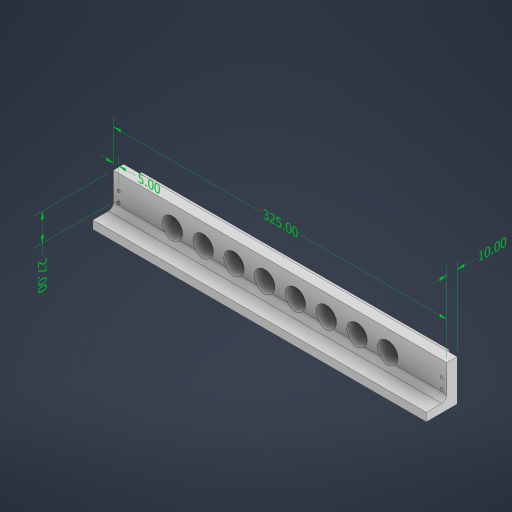
# Autodesk Inventor part: chessboard-base-1
Saved by Autodesk Inventor 2023 (Build 270158000, 158)
## iProperties
Created: 2023-12-20
Part Number: chessboard-base-1
Material: Generic
Document SubType Name: Modeling
Designer: hrush
Density: 1 g/cm^3
Appearance: Default
Author: hrush
Autodesk Inventor part; units mm, degrees
ref_plane "YZ Plane" through (0, 0, 0) normal (1, 0, 0) x (0, 1, 0)
ref_plane "XZ Plane" through (0, 0, 0) normal (0, 1, 0) x (-1, 0, 0)
ref_plane "XY Plane" through (0, 0, 0) normal (0, 0, 1) x (1, 0, 0)
sketch "Sketch1" plane through (0, 0, 0) normal (0, 1, 0) x (-1, 0, 0)
  line L0 (0, 0) -> (325, 0)
  line L1 (325, 0) -> (325, -10)
  line L2 (325, -10) -> (0, -10)
  line L3 (0, -10) -> (0, 0)
  dimension "d0" = 325
  dimension "d1" = 10
  constraints: 8 end point, 2 parallel, 1 horizontal, 1 perpendicular
  measures "d0" distance of L1.end L2.end
  measures "d1" distance of L0.end L1.end
extrude "Extrusion1" add sketch "Sketch1" along normal blind 40
sketch "Sketch4" plane through (-325, 0, 0) normal (0, 0, 1) x (1, 0, 0)
  line L0 (325, 0) -> (0, 0) projected
  line L1 (325, 0) -> (325, 40) projected
  line L2 (0, 0) -> (325, 0)
  line L3 (325, 0) -> (325, 8)
  line L4 (325, 8) -> (0, 8)
  line L5 (0, 8) -> (0, 0)
  dimension "d34" = 8
  constraints: 8 end point, 2 parallel, 1 horizontal, 1 perpendicular, 1 point on line
  measures "d34" distance of L3.end L2.end
extrude "Extrusion3" add sketch "Sketch4" along normal blind 20
sketch "Sketch5" plane through (-325, 40, 0) normal (0, 0, 1) x (1, 0, 0)
  circle A0 centre (320, -25) radius 1.5
  circle A1 centre (320, -15) radius 1.5
  line L0 (325, -32) -> (325, 0) projected
  line L1 (0, 0) -> (325, 0) projected
  circle A2 centre (5, -15) radius 1.5
  circle A3 centre (5, -25) radius 1.5
  line L2 (0, -32) -> (0, 0) projected
  point P0 (325, -40)
  point P1 (325, -27)
  point P2 (0, -27)
  dimension "d39" = 3
  dimension "d40" = 3
  dimension "d41" = 5
  dimension "d42" = 5
  dimension "d43" = 10
  dimension "d44" = 15
  dimension "d45" = 3
  dimension "d46" = 3
  dimension "d47" = 10
  dimension "d48" = 15
  dimension "d49" = 5
  dimension "d50" = 5
  constraints: 4 centre point
  measures "d39" diameter of A0
  measures "d40" diameter of A1
  measures "d41" distance from line of L0 A0.centre
  measures "d42" distance from line of L0 A1.centre
  measures "d43" distance of A0.centre A1.centre
  measures "d44" distance from line of L1 A1.centre
  measures "d45" diameter of A2
  measures "d46" diameter of A3
  measures "d47" distance of A2.centre A3.centre
  measures "d48" distance from line of L1 A2.centre
  measures "d49" distance from line of L2 A2.centre
  measures "d50" distance from line of L2 A3.centre
extrude "Extrusion4" cut sketch "Sketch5" against normal blind 20
thread "Thread1" size "M3x0.5" class "6H" standard "ANSI Metric M Profile" full length
thread "Thread2" size "M3x0.5" class "6H" standard "ANSI Metric M Profile" full length
thread "Thread3" size "M3x0.5" class "6H" standard "ANSI Metric M Profile" full length
thread "Thread4" size "M3x0.5" class "6H" standard "ANSI Metric M Profile" full length
sketch "Sketch8" plane through (0, 0, -10) normal (0, 0, -1) x (-1, 0, 0)
  line L0 (0, 40) -> (325, 40) projected
  line L1 (12.5, 37) -> (312.5, 37)
  line L2 (312.5, 37) -> (312.5, 0)
  line L3 (312.5, 0) -> (12.5, 0)
  line L4 (12.5, 0) -> (12.5, 37)
  line L5 (0, 0) -> (0, 40) projected
  line L6 (325, 0) -> (325, 40) projected
  point P0 (312.5, 18.5)
  dimension "d67" = 300
  dimension "d68" = 37
  dimension "d69" = 12.5
  dimension "d70" = 12.5
  dimension "d71" = 3
  constraints: 8 end point, 2 parallel, 1 horizontal, 1 midpoint, 1 perpendicular
  measures "d67" distance of L2.end L3.end
  measures "d68" distance of L1.end L2.end
  measures "d69" distance from line of L5 L1.start
  measures "d70" distance from line of L6 point (312.5, 18.5)
  measures "d71" distance between parallel lines of L0 L1
extrude "Extrusion5" add sketch "Sketch8" along normal blind 5
sketch "Sketch9" plane through (-325, 40, 0) normal (0, 0, 1) x (1, 0, 0)
  circle A0 centre (57.4993, -19.9899) radius 10
  circle A1 centre (87.4993, -19.9899) radius 10
  circle A2 centre (117.4993, -19.9899) radius 10
  circle A3 centre (147.4993, -19.9899) radius 10
  circle A4 centre (177.4993, -19.9899) radius 10
  circle A5 centre (207.4993, -19.9899) radius 10
  circle A6 centre (237.4993, -19.9899) radius 10
  circle A7 centre (267.4993, -19.9899) radius 10
  line L0 (-0.0007, -39.9899) -> (-0.0007, 0.0101)
  line L1 (324.9993, -39.9899) -> (324.9993, 0.0101)
  line L2 (-0.0007, 0.0101) -> (324.9993, 0.0101)
  point P0 (325, -40)
  dimension "d74" = 20
  dimension "d75" = 20
  dimension "d76" = 20
  dimension "d77" = 20
  dimension "d78" = 20
  dimension "d79" = 20
  dimension "d80" = 20
  dimension "d81" = 20
  dimension "d82" = 30
  dimension "d83" = 30
  dimension "d84" = 30
  dimension "d85" = 30
  dimension "d86" = 30
  dimension "d87" = 30
  dimension "d88" = 30
  dimension "d89" = 57.5
  dimension "d90" = 20
  dimension "d91" = 57.5
  constraints: 8 centre point, 6 end point
  measures "d74" diameter of A0
  measures "d75" diameter of A1
  measures "d76" diameter of A2
  measures "d77" diameter of A3
  measures "d78" diameter of A4
  measures "d79" diameter of A5
  measures "d80" diameter of A6
  measures "d81" diameter of A7
  measures "d82" distance of A0.centre A1.centre
  measures "d83" distance of A1.centre A2.centre
  measures "d84" distance of A2.centre A3.centre
  measures "d85" distance of A3.centre A4.centre
  measures "d86" distance of A4.centre A5.centre
  measures "d87" distance of A5.centre A6.centre
  measures "d88" distance of A6.centre A7.centre
  measures "d89" distance from line of L1 A7.centre
  measures "d90" distance from line of L2 A0.centre
  measures "d91" distance from line of L0 A0.centre
extrude "Extrusion6" cut sketch "Sketch9" against normal blind 40
fillet "Fillet2" radius 5 1 edges at (-162.5, 8, 0)
equation "\"d83\" = d82"
equation "\"d84\" = d83"
equation "\"d85\" = d84"
equation "\"d86\" = d85"
equation "\"d87\" = d86"
equation "\"d88\" = d87"
body "Solid1"
